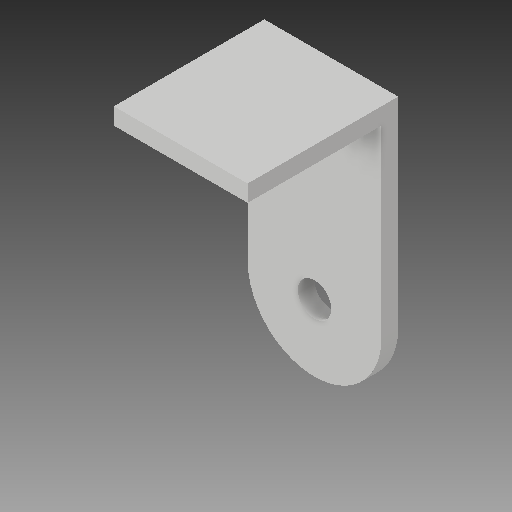
# Autodesk Inventor part: Roller holder
Saved by Autodesk Inventor 2017 (Build 210142000, 142)
## iProperties
Created: 2019-02-07
Part Number: Roller holder
Material: Generic
Document SubType Name: Modeling
Designer: S346795925
Density: 1 g/cm^3
Appearance: Default
Author: S346795925
Autodesk Inventor part; units mm, degrees
ref_plane "YZ Plane" through (0, 0, 0) normal (1, 0, 0) x (0, 1, 0)
ref_plane "XZ Plane" through (0, 0, 0) normal (0, 1, 0) x (-1, 0, 0)
ref_plane "XY Plane" through (0, 0, 0) normal (0, 0, 1) x (1, 0, 0)
sketch "Sketch1" plane through (0, 0, 0) normal (0, 0, 1) x (1, 0, 0)
  circle A0 centre (0, 0) radius 12.7
  line L0 (12.7, 0) -> (12.7, 38.1)
  line L1 (-12.7, 0) -> (-12.7, 38.1)
  line L2 (-12.7, 38.1) -> (12.7, 38.1)
  circle A1 centre (0, 0) radius 3.175
  dimension "d0" = 25.4
  dimension "d1" = 38.1
  dimension "d3" = 6.35
  constraints: 6 end point, 2 centre point, 2 coincident, 2 point on circle, 2 tangent, 2 vertical
  measures "d0" diameter of A0
  measures "d1" distance of L0.start L0.end
  measures "d3" diameter of A1
extrude "Extrusion1" add sketch "Sketch1" along normal blind 3.175
sketch "Sketch2" plane through (0, 0, 3.175) normal (0, 0, 1) x (1, 0, 0)
  line L0 (12.7, 38.1) -> (-12.7, 38.1) projected
  line L1 (-12.7, 38.1) -> (12.7, 38.1)
  line L2 (12.7, 38.1) -> (12.7, 34.925)
  line L3 (12.7, 34.925) -> (-12.7, 34.925)
  line L4 (-12.7, 34.925) -> (-12.7, 38.1)
  point P0 (0, 0)
  dimension "d6" = 25.4
  dimension "d7" = 3.175
  constraints: 8 end point, 2 parallel, 1 horizontal, 1 perpendicular
  measures "d6" distance of L2.end L3.end
  measures "d7" distance of L1.end L2.end
extrude "Extrusion2" add sketch "Sketch2" along normal blind 25.4
body "Solid1"
